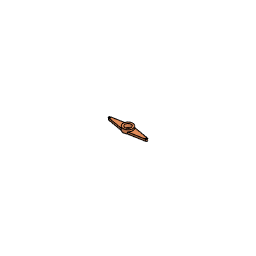
prototype v2 v10 (Autodesk Fusion 360 archive; units mm, degrees)
design "servo_wing"
Autodesk Fusion 360 part; units mm, degrees
sketch "Sketch1" plane through (0, 0, -16) normal (0, 0, -1) x (1, 0, 0)
  arc A0 (-4.6411, 2.2588) -> (-4.984, 2.469) centre (-5.0864, 1.9172) ccw
  arc A1 (-4.984, 2.469) -> (-5.375, 2.375) centre (-5.057, 1.9125) ccw
  arc A2 (-5.375, 2.375) -> (-5.766, 2.469) centre (-5.693, 1.9125) ccw
  arc A3 (-5.766, 2.469) -> (-6.1089, 2.2588) centre (-5.6636, 1.9172) ccw
  arc A4 (-6.1089, 2.2588) -> (-6.5099, 2.2273) centre (-6.2684, 1.7206) ccw
  arc A5 (-6.5099, 2.2273) -> (-6.771, 1.9214) centre (-6.2419, 1.7341) ccw
  arc A6 (-6.771, 1.9214) -> (-7.1426, 1.7676) centre (-6.7564, 1.3604) ccw
  arc A7 (-7.1426, 1.7676) -> (-7.2964, 1.396) centre (-6.7354, 1.3814) ccw
  arc A8 (-7.2964, 1.396) -> (-7.6023, 1.1349) centre (-7.1091, 0.8669) ccw
  arc A9 (-7.6023, 1.1349) -> (-7.6338, 0.7339) centre (-7.0956, 0.8934) ccw
  arc A10 (-7.6338, 0.7339) -> (-7.844, 0.391) centre (-7.2921, 0.2886) ccw
  arc A11 (-7.844, 0.391) -> (-7.75, 0) centre (-7.2875, 0.318) ccw
  arc A12 (-7.75, 0) -> (-7.844, -0.391) centre (-7.2875, -0.318) ccw
  arc A13 (-7.844, -0.391) -> (-7.6338, -0.7339) centre (-7.2921, -0.2886) ccw
  arc A14 (-7.6338, -0.7339) -> (-7.6023, -1.1349) centre (-7.0956, -0.8934) ccw
  arc A15 (-7.6023, -1.1349) -> (-7.2964, -1.396) centre (-7.1091, -0.8669) ccw
  arc A16 (-7.2964, -1.396) -> (-7.1426, -1.7676) centre (-6.7354, -1.3814) ccw
  arc A17 (-7.1426, -1.7676) -> (-6.771, -1.9214) centre (-6.7564, -1.3604) ccw
  arc A18 (-6.771, -1.9214) -> (-6.5099, -2.2273) centre (-6.2419, -1.7341) ccw
  arc A19 (-6.5099, -2.2273) -> (-6.1089, -2.2588) centre (-6.2684, -1.7206) ccw
  arc A20 (-6.1089, -2.2588) -> (-5.766, -2.469) centre (-5.6636, -1.9171) ccw
  arc A21 (-5.766, -2.469) -> (-5.375, -2.375) centre (-5.693, -1.9125) ccw
  arc A22 (-5.375, -2.375) -> (-4.984, -2.469) centre (-5.057, -1.9125) ccw
  arc A23 (-4.984, -2.469) -> (-4.6411, -2.2588) centre (-5.0864, -1.9171) ccw
  arc A24 (-4.6411, -2.2588) -> (-4.2401, -2.2273) centre (-4.4816, -1.7206) ccw
  arc A25 (-4.2401, -2.2273) -> (-3.979, -1.9214) centre (-4.5081, -1.7341) ccw
  arc A26 (-3.979, -1.9214) -> (-3.6074, -1.7676) centre (-3.9936, -1.3604) ccw
  arc A27 (-3.6074, -1.7676) -> (-3.4536, -1.396) centre (-4.0146, -1.3814) ccw
  arc A28 (-3.4536, -1.396) -> (-3.1477, -1.1349) centre (-3.6409, -0.8669) ccw
  arc A29 (-3.1477, -1.1349) -> (-3.1162, -0.7339) centre (-3.6544, -0.8934) ccw
  arc A30 (-3.1162, -0.7339) -> (-2.906, -0.391) centre (-3.4579, -0.2886) ccw
  arc A31 (-2.906, -0.391) -> (-3, 0) centre (-3.4625, -0.318) ccw
  arc A32 (-3, 0) -> (-2.906, 0.391) centre (-3.4625, 0.318) ccw
  arc A33 (-2.906, 0.391) -> (-3.1162, 0.7339) centre (-3.4579, 0.2886) ccw
  arc A34 (-3.1162, 0.7339) -> (-3.1477, 1.1349) centre (-3.6544, 0.8934) ccw
  arc A35 (-3.1477, 1.1349) -> (-3.4536, 1.396) centre (-3.6409, 0.8669) ccw
  arc A36 (-3.4536, 1.396) -> (-3.6074, 1.7676) centre (-4.0146, 1.3814) ccw
  arc A37 (-3.6074, 1.7676) -> (-3.979, 1.9214) centre (-3.9936, 1.3604) ccw
  arc A38 (-3.979, 1.9214) -> (-4.2401, 2.2273) centre (-4.5081, 1.7341) ccw
  arc A39 (-4.2401, 2.2273) -> (-4.6411, 2.2588) centre (-4.4816, 1.7206) ccw
  circle A40 centre (-5.375, 0) radius 1.5
  circle A41 centre (-5.375, 0) radius 1.2295
  circle A42 centre (-5.375, 0) radius 2.5
  circle A43 centre (-5.375, 0) radius 4
  line L0 (-5.375, 0) -> (-5.375, -4) construction
  line L1 (-5.375, 0) -> (-5.375, 4) construction
  line L2 (-5.375, 0) -> (-2.8038, -3.0642) construction
  line L3 (-5.375, 0) -> (-1.375, 0) construction
  line L4 (-5.375, 0) -> (-2.8038, 3.0642) construction
  line L5 (-5.375, 0) -> (-1.375, 0) construction
  line L6 (-5.375, 0) -> (-7.9462, -3.0642) construction
  line L7 (-5.375, 0) -> (-7.9462, 3.0642) construction
  line L8 (-5.375, 0) -> (14.625, 0) construction
  line L9 (-5.375, 0) -> (-25.375, 0) construction
  line L10 (-7.9462, -3.0642) -> (-25.375, 0)
  line L11 (-25.375, 0) -> (-7.9462, 3.0642)
  line L12 (14.625, 0) -> (-2.8038, -3.0642)
  line L13 (-2.8038, 3.0642) -> (14.625, 0)
  line L14 (14.625, 0) -> (9.625, 0) construction
  line L15 (-25.375, 0) -> (-20.375, 0) construction
  circle A44 centre (-20.375, 0) radius 0.5
  circle A45 centre (9.625, 0) radius 0.5
  dimension "d346" = 5
  dimension "d347" = 8
  dimension "d348" = 50
  dimension "d349" = 50
  dimension "d350" = 20
  dimension "d351" = 20
  dimension "d352" = 5
  dimension "d353" = 5
  dimension "d354" = 1
  dimension "d355" = 1
  constraint concentric A40 A42
  constraint concentric A40 A43
  constraint coincident A40.centre A41.centre
  constraint coincident A43 L0.end
  constraint vertical L0
  constraint coincident A43 L1.end
  constraint parallel L0 L1
  constraint horizontal L3
  constraint horizontal L5
  constraint coincident A43 L6.end
  constraint coincident A43 L7.end
  constraint perpendicular L0 L8
  constraint horizontal L9
  constraint parallel L8 L14
  constraint parallel L9 L15
  constraint coincident L15.end A44.centre
  constraint coincident L14.end A45.centre
  measures "d346" diameter of A42
  measures "d347" diameter of A43
  measures "d348" angle of L2 L3
  measures "d349" angle of L4 L5
  measures "d350" distance of A40.centre L8.end
  measures "d351" distance of A40.centre L9.end
  measures "d352" distance of L8.end L14.end
  measures "d353" distance of L9.end L15.end
  measures "d354" diameter of A44
  measures "d355" diameter of A45
extrude "Extrude1" add sketch "Sketch1" against normal blind 3 contours A43
extrude "Extrude2" add sketch "Sketch1" against normal blind 1.5 contours A43 L12 L13 | A43 L10 L11
fillet "Fillet1" radius 0.8 2 edges at (-25.375, 0, -15.25) (14.625, 0, -15.25)

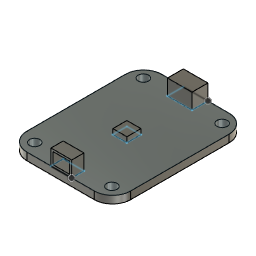
design "BME680"
Autodesk Fusion 360 part; units mm, degrees
sketch "Sketch1" plane through (0, 0, 0) normal (0, 0, 1) x (1, 0, 0)
  line L0 (10, 13) -> (-10, 13)
  line L1 (-10, 13) -> (-10, -13)
  line L2 (-10, -13) -> (10, -13)
  line L3 (10, -13) -> (10, 13)
  line L4 (10, 13) -> (-10, -13) construction
  line L5 (-10, 13) -> (10, -13) construction
  dimension "d1" = 20
  dimension "d2" = 26
  constraint horizontal L0
  constraint perpendicular L0 L1
  constraint parallel L0 L2
  constraint parallel L1 L3
  constraint coincident L4 origin
  constraint coincident L5 origin
  measures "d1" distance of L1.end L2.end
  measures "d2" distance of L0.end L1.end
extrude "Extrude1" add sketch "Sketch1" along normal blind 1.45 makes body 1
fillet "Fillet1" radius 3.5 4 edges at (10, 13, 0.725) (10, -13, 0.725) (-10, -13, 0.725) (-10, 13, 0.725) on bodies 1
hole "Hole1" at (7.531, 10.6352, 1.45) direction (0, 0, -1) diameter 2 depth 6 tip angle 118 bodies 1
hole "Hole2" at (-7.6326, 10.5966, 1.45) direction (0, 0, -1) diameter 2 depth 6 tip angle 118 bodies 1
hole "Hole3" at (7.415, -10.5242, 1.45) direction (0, 0, -1) diameter 2 depth 6 tip angle 118 bodies 1
hole "Hole4" at (-7.3618, -10.6402, 1.45) direction (0, 0, -1) diameter 2 depth 6 tip angle 118 bodies 1
sketch "Sketch2" plane through (0, 0, 1.45) normal (0, 0, 1) x (-1, 0, 0)
  circle A0 centre (7.3618, 10.6402) radius 1
  circle A1 centre (-7.415, 10.5242) radius 1
  circle A2 centre (7.6326, -10.5966) radius 1
  circle A3 centre (-7.531, -10.6352) radius 1
  arc A4 (6.5, -13) -> (10, -9.5) centre (6.5, -9.5) ccw
  line L0 (10, -9.5) -> (10, 9.5)
  arc A5 (10, 9.5) -> (6.5, 13) centre (6.5, 9.5) ccw
  line L1 (6.5, 13) -> (-6.5, 13)
  arc A6 (-6.5, 13) -> (-10, 9.5) centre (-6.5, 9.5) ccw
  line L2 (-10, 9.5) -> (-10, -9.5)
  arc A7 (-10, -9.5) -> (-6.5, -13) centre (-6.5, -9.5) ccw
  line L3 (-6.5, -13) -> (6.5, -13)
  line L4 (-1.576, 1.7941) -> (1.1396, 1.7941)
  line L5 (1.1396, 1.7941) -> (1.1396, -0.9214)
  line L6 (1.1396, -0.9214) -> (-1.576, -0.9214)
  line L7 (-1.576, -0.9214) -> (-1.576, 1.7941)
  line L8 (-2.133, 13) -> (1.8707, 13)
  line L9 (1.8707, 13) -> (1.8707, 10.637)
  line L10 (1.8707, 10.637) -> (-2.133, 10.637)
  line L11 (-2.133, 10.637) -> (-2.133, 13)
  line L12 (-2.4115, -13) -> (2.3232, -13)
  line L13 (2.3232, -13) -> (2.3232, -9.9383)
  line L14 (2.3232, -9.9383) -> (-2.4115, -9.9383)
  line L15 (-2.4115, -9.9383) -> (-2.4115, -13)
  constraint horizontal L4
  constraint vertical L5
  constraint horizontal L6
  constraint vertical L7
  constraint horizontal L8
  constraint vertical L9
  constraint horizontal L10
  constraint vertical L11
  constraint coincident L1 L8.start
  constraint horizontal L12
  constraint vertical L13
  constraint horizontal L14
  constraint vertical L15
  constraint coincident L3 L12.start
extrude "Extrude2" add sketch "Sketch2" along normal blind 1 contours L4 L5 L6 L7 bodies 1
extrude "Extrude3" add sketch "Sketch2" along normal blind 3 separate body contours L3 L12 L13 L14 L15 | L1 L8 L9 L10 L11 makes body 2 at (-0.5361, -10.637, 2.45) makes body 3 at (-0.745, 11.9794, 1.45)
shell "Shell1" thickness 0.4 removed faces 1 at (-0.5361, -13, 2.45) on bodies 2
shell "Shell2" thickness 0.4 removed faces 1 at (0.8333, 13, 2.45) on bodies 3

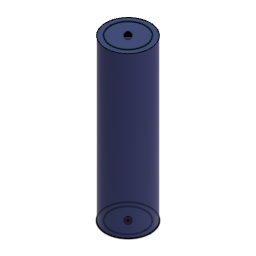
design "Li-ion 18-650"
Autodesk Fusion 360 part; units mm, degrees
sketch "Sketch1" plane through (0, 0, 0) normal (0, 0, 1) x (1, 0, 0)
  circle A0 centre (0, 0) radius 9
  circle A1 centre (0, 0) radius 7
  dimension "d1" = 18
  dimension "d2" = 14
  constraint coincident A0.centre A1.centre
  constraint concentric A0 A1
  measures "d1" diameter of A0
  measures "d2" diameter of A1
extrude "Extrude1" add sketch "Sketch1" along normal blind 65 contours A0 | A1
sketch "Sketch2" plane through (0, 0, 65) normal (0, 0, 1) x (-1, 0, 0)
  circle A0 centre (0, 0) radius 9
  circle A1 centre (0, 0) radius 7
  dimension "d5" = 14
  constraint coincident A0.centre A1.centre
  measures "d5" diameter of A1

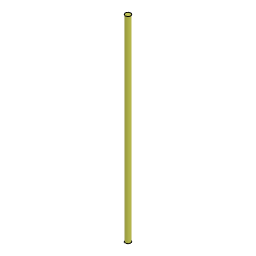
design "threaded_bolt"
Autodesk Fusion 360 part; units mm, degrees
sketch "Sketch1" plane through (0, 0, 0) normal (0, 0, 1) x (1, 0, 0)
  circle A0 centre (0, 0) radius 1.4
  dimension "d190" = 2.8
  constraint coincident A0.centre origin
  measures "d190" diameter of A0
extrude "Extrude1" add sketch "Sketch1" along normal blind 115
move_face "OffsetFaces1" offset -5 4 faces at (0.5063, -0.2629, 0) (0.5063, -0.2629, 0) (0.5063, -0.2629, 0) (0.5063, -0.2629, 0)
thread "Thread1" "ISO Metric profile 3.0 M3x0.5 6g" major diameter 2.927 minor diameter 2.3555 pitch 0.5 angle 60 resizes the face on face at (1.3981, 0.0733, 41.6667)
